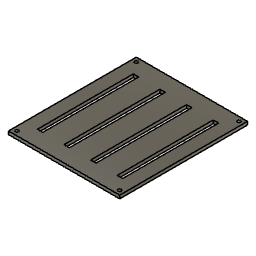
Quadrotor_controller_case_lid_plain (Autodesk Fusion 360 design; units mm, degrees)
Autodesk Fusion 360 part; units mm, degrees
sketch "Sketch1" plane through (0, 0, 0) normal (0, 0, 1) x (1, 0, 0)
  line L0 (-52.2, -60) -> (52.2, -60)
  line L1 (52.2, -60) -> (52.2, 60)
  line L2 (52.2, 60) -> (-52.2, 60)
  line L3 (-52.2, 60) -> (-52.2, -60)
  dimension "d1" = 104.4
  dimension "d2" = 120
  dimension "d3" = 60
  dimension "d4" = 52.2
  constraint horizontal L0
  constraint vertical L1
  constraint horizontal L2
  constraint vertical L3
  measures "d1" distance of L0.start L0.end
  measures "d2" distance of L0.start L2.end
  measures "d3" vertical distance of origin L0.start
  measures "d4" horizontal distance of origin L0.start
extrude "Extrude1" add sketch "Sketch1" along normal blind 3
sketch "Sketch2" plane through (0, 0, 3) normal (0, 0, 1) x (-1, 0, 0)
  line L0 (52.2, -60) -> (52.2, 60)
  line L1 (52.2, 60) -> (-52.2, 60)
  line L2 (-52.2, 60) -> (-52.2, -60)
  line L3 (-52.2, -60) -> (52.2, -60)
  circle A0 centre (-48.2, -56) radius 1.5
  circle A1 centre (48.2, -56) radius 1.5
  circle A2 centre (48.2, 56) radius 1.5
  circle A3 centre (-48.2, 56) radius 1.5
  dimension "d7" = 3
  dimension "d8" = 3
  dimension "d9" = 3
  dimension "d10" = 3
  dimension "d11" = 4
  dimension "d12" = 4
  dimension "d13" = 4
  dimension "d14" = 4
  dimension "d15" = 4
  dimension "d16" = 4
  dimension "d17" = 4
  dimension "d18" = 4
  measures "d7" diameter of A0
  measures "d8" diameter of A1
  measures "d9" diameter of A3
  measures "d10" diameter of A2
  measures "d11" distance of L2 A0.centre
  measures "d12" distance of L3 A0.centre
  measures "d13" distance of L3 A1.centre
  measures "d14" distance of L0 A1.centre
  measures "d15" distance of L1 A2.centre
  measures "d16" distance of L0 A2.centre
  measures "d17" distance of L2 A3.centre
  measures "d18" distance of L1 A3.centre
hole "Hole1" at (-48.2, 56, 3) at (48.2, 56, 3) at (48.2, -56, 3) at (-48.2, -56, 3) direction (0, 0, -1) diameter 3 depth 3 tip angle 118
sketch "Sketch4" plane through (0, 0, 3) normal (0, 0, 1) x (-1, 0, 0)
  circle A0 centre (-48.2, 56) radius 1.5
  circle A1 centre (48.2, -56) radius 1.5
  circle A2 centre (-48.2, -56) radius 1.5
  circle A3 centre (48.2, 56) radius 1.5
  line L0 (52.2, -60) -> (52.2, 60)
  line L1 (52.2, 60) -> (-52.2, 60)
  line L2 (-52.2, 60) -> (-52.2, -60)
  line L3 (-52.2, -60) -> (52.2, -60)
  line L4 (40, -45) -> (35, -45)
  line L5 (35, -45) -> (35, 45)
  line L6 (35, 45) -> (40, 45)
  line L7 (40, 45) -> (40, -45)
  line L8 (10, -45) -> (10, 45)
  line L9 (10, 45) -> (15, 45)
  line L10 (15, 45) -> (15, -45)
  line L11 (15, -45) -> (10, -45)
  line L12 (-15, -45) -> (-15, 45)
  line L13 (-15, 45) -> (-10, 45)
  line L14 (-10, 45) -> (-10, -45)
  line L15 (-10, -45) -> (-15, -45)
  line L16 (-40, -45) -> (-40, 45)
  line L17 (-40, 45) -> (-35, 45)
  line L18 (-35, 45) -> (-35, -45)
  line L19 (-35, -45) -> (-40, -45)
  dimension "d39" = -75
  dimension "d40" = 0
  dimension "d41" = 5
  dimension "d42" = 90
  dimension "d43" = 40
  dimension "d44" = 45
  constraint horizontal L4
  constraint vertical L5
  constraint horizontal L6
  constraint vertical L7
  measures "d41" distance of L4.start L4.end
  measures "d42" distance of L4.start L6.end
  measures "d43" distance of origin L7
  measures "d44" distance of origin L4
extrude "Extrude2" cut sketch "Sketch4" against normal blind 3 contours L4 L5 L6 L7 | L8 L9 L10 L11 | L12 L13 L14 L15 | L16 L17 L18 L19
sketch "Sketch6" plane through (0, 0, 3) normal (0, 0, 1) x (-1, 0, 0)
  line L0 (10, 45) -> (15, 45)
  line L1 (15, 45) -> (15, -45)
  line L2 (15, -45) -> (10, -45)
  line L3 (10, -45) -> (10, 45)
  line L4 (-15, 45) -> (-10, 45)
  line L5 (-10, 45) -> (-10, -45)
  line L6 (-10, -45) -> (-15, -45)
  line L7 (-15, -45) -> (-15, 45)
  line L8 (35, -45) -> (35, 45)
  line L9 (35, 45) -> (40, 45)
  line L10 (40, 45) -> (40, -45)
  line L11 (40, -45) -> (35, -45)
  line L12 (-40, 45) -> (-35, 45)
  line L13 (-35, 45) -> (-35, -45)
  line L14 (-35, -45) -> (-40, -45)
  line L15 (-40, -45) -> (-40, 45)
  circle A0 centre (-48.2, 56) radius 1.5
  circle A1 centre (48.2, -56) radius 1.5
  circle A2 centre (-48.2, -56) radius 1.5
  circle A3 centre (48.2, 56) radius 1.5
  line L16 (52.2, -60) -> (52.2, 60)
  line L17 (52.2, 60) -> (-52.2, 60)
  line L18 (-52.2, 60) -> (-52.2, -60)
  line L19 (-52.2, -60) -> (52.2, -60)
  line L20 (-15, 25) -> (15, 25)
  line L21 (15, 25) -> (15, -25)
  line L22 (15, -25) -> (-15, -25)
  line L23 (-15, -25) -> (-15, 25)
  line L24 (-15, 25) -> (15, -25) construction
  line L25 (15, 25) -> (-15, -25) construction
  line L26 (40, -8) -> (35, -8)
  line L27 (35, -8) -> (35, 8)
  line L28 (35, 8) -> (40, 8)
  line L29 (40, 8) -> (40, -8)
  line L30 (-35, -8) -> (-40, -8)
  line L31 (-40, -8) -> (-40, 8)
  line L32 (-40, 8) -> (-35, 8)
  line L33 (-35, 8) -> (-35, -8)
  dimension "d49" = 50
  dimension "d56" = 8
  dimension "d57" = 16
  dimension "d58" = 8
  dimension "d59" = 16
  constraint horizontal L20
  constraint perpendicular L20 L21
  constraint parallel L20 L22
  constraint parallel L21 L23
  constraint coincident L24 origin
  constraint coincident L25 origin
  constraint coincident L7 L20.start
  constraint horizontal L26
  constraint vertical L27
  constraint horizontal L28
  constraint vertical L29
  constraint coincident L8 L27.end
  constraint coincident L10 L26.start
  constraint horizontal L30
  constraint vertical L31
  constraint horizontal L32
  constraint vertical L33
  constraint coincident L15 L31.end
  constraint coincident L13 L30.start
  measures "d49" distance of L20.end L21.end
  measures "d56" vertical distance of origin L27.end
  measures "d57" vertical distance of L26.start L27.end
  measures "d58" vertical distance of origin L31.end
  measures "d59" vertical distance of L30.start L31.end
extrude "Extrude3" [rolled back] along distance -3 taper angle 0
sketch "Sketch5" plane through (0, 0, 3) normal (0, 0, 1) x (-1, 0, 0)
  line L0 (10, 45) -> (15, 45)
  line L1 (15, 45) -> (15, 25)
  line L2 (15, -45) -> (10, -45)
  line L3 (10, 25) -> (10, 45)
  line L4 (-15, 45) -> (-10, 45)
  line L5 (-10, -25) -> (-10, -45)
  line L6 (-10, -45) -> (-15, -45)
  line L7 (-15, -45) -> (-15, -25)
  line L8 (35, 8) -> (35, 45)
  line L9 (35, 45) -> (40, 45)
  line L10 (40, 45) -> (40, 8)
  line L11 (40, -45) -> (35, -45)
  line L12 (-40, 45) -> (-35, 45)
  line L13 (-35, 45) -> (-35, 8)
  line L14 (-35, -45) -> (-40, -45)
  line L15 (-40, 8) -> (-40, 45)
  circle A0 centre (-48.2, 56) radius 1.5
  circle A1 centre (48.2, -56) radius 1.5
  circle A2 centre (-48.2, -56) radius 1.5
  circle A3 centre (48.2, 56) radius 1.5
  line L16 (52.2, -60) -> (52.2, 60)
  line L17 (52.2, 60) -> (-52.2, 60)
  line L18 (-52.2, 60) -> (-52.2, -60)
  line L19 (-52.2, -60) -> (52.2, -60)
  circle A4 centre (0, 0) radius 11.25
  circle A5 centre (0, 0) radius 15
  line L20 (15, 25) -> (10, 25)
  line L21 (-15, -25) -> (-10, -25)
  line L22 (10, -25) -> (15, -25)
  line L23 (15, -25) -> (15, -45)
  line L24 (10, -45) -> (10, -25)
  line L25 (-10, 25) -> (-15, 25)
  line L26 (-15, 25) -> (-15, 45)
  line L27 (-10, 45) -> (-10, 25)
  line L28 (-35, 8) -> (-40, 8)
  line L29 (40, 8) -> (35, 8)
  line L30 (35, -8) -> (40, -8)
  line L31 (40, -8) -> (40, -45)
  line L32 (35, -45) -> (35, -8)
  line L33 (-40, -8) -> (-35, -8)
  line L34 (-35, -8) -> (-35, -45)
  line L35 (-40, -45) -> (-40, -8)
  dimension "d47" = 22.5
  dimension "d48" = 30
  constraint coincident A4.centre A5.centre
  measures "d47" diameter of A4
  measures "d48" diameter of A5
extrude "Extrude4" [rolled back] along distance 30 taper angle 0
fillet "Fillet1" [rolled back] radius 6
chamfer "Chamfer1" [rolled back] distance 0.5
sketch "Sketch7" plane through (0, 0, 0) normal (0, 1, 0) x (1, 0, 0)
  circle A0 centre (-0.0436, -26) radius 1.5
  dimension "d61" = 26
  dimension "d62" = 3
  measures "d61" vertical distance of origin A0.centre
  measures "d62" diameter of A0
hole "Hole3" [rolled back] hole depth 17 hole diameter 3 tip angle 118
thread "Thread1" [rolled back]
pattern_circular "C-Pattern1" [rolled back] total angle 360
hole "Hole4" [rolled back] hole depth 3 hole diameter 16 tip angle 118
sketch "Sketch8" plane through (0, 0, 0) normal (0, 0, -1) x (1, 0, 0)
  circle A0 centre (0, 0) radius 8
  line L0 (40, -8) -> (40, -45)
  line L1 (40, -45) -> (35, -45)
  line L2 (35, -45) -> (35, -8)
  line L3 (35, -8) -> (40, -8)
  line L4 (-10, -25) -> (-10, -45)
  line L5 (-10, -45) -> (-15, -45)
  line L6 (-15, -45) -> (-15, -25)
  line L7 (-15, -25) -> (-10, -25)
  line L8 (-35, -8) -> (-35, -45)
  line L9 (-35, -45) -> (-40, -45)
  line L10 (-40, -45) -> (-40, -8)
  line L11 (-40, -8) -> (-35, -8)
  line L12 (10, 25) -> (10, 45)
  line L13 (10, 45) -> (15, 45)
  line L14 (15, 45) -> (15, 25)
  line L15 (15, 25) -> (10, 25)
  line L16 (-10, 25) -> (-15, 25)
  line L17 (-15, 25) -> (-15, 45)
  line L18 (-15, 45) -> (-10, 45)
  line L19 (-10, 45) -> (-10, 25)
  line L20 (10, -25) -> (15, -25)
  line L21 (15, -25) -> (15, -45)
  line L22 (15, -45) -> (10, -45)
  line L23 (10, -45) -> (10, -25)
  line L24 (-35, 8) -> (-40, 8)
  line L25 (-40, 8) -> (-40, 45)
  line L26 (-40, 45) -> (-35, 45)
  line L27 (-35, 45) -> (-35, 8)
  line L28 (40, 8) -> (35, 8)
  line L29 (35, 8) -> (35, 45)
  line L30 (35, 45) -> (40, 45)
  line L31 (40, 45) -> (40, 8)
  circle A1 centre (48.2, 56) radius 1.5
  circle A2 centre (-48.2, -56) radius 1.5
  circle A3 centre (48.2, -56) radius 1.5
  circle A4 centre (-48.2, 56) radius 1.5
  line L32 (-52.2, 60) -> (-52.2, -60)
  line L33 (-52.2, -60) -> (52.2, -60)
  line L34 (52.2, -60) -> (52.2, 60)
  line L35 (52.2, 60) -> (-52.2, 60)
  line L36 (-21.595, 55.595) -> (21.595, 55.595)
  line L37 (21.595, 55.595) -> (21.595, 12.405)
  line L38 (21.595, 12.405) -> (-21.595, 12.405)
  line L39 (-21.595, 12.405) -> (-21.595, 55.595)
  line L40 (-25.4, -12.405) -> (25.4, -12.405)
  line L41 (25.4, -12.405) -> (25.4, -55.595)
  line L42 (25.4, -55.595) -> (-25.4, -55.595)
  line L43 (-25.4, -55.595) -> (-25.4, -12.405)
  line L44 (-19.055, 53.055) -> (19.055, 53.055)
  line L45 (19.055, 53.055) -> (19.055, 14.945)
  line L46 (19.055, 14.945) -> (-19.055, 14.945)
  line L47 (-19.055, 14.945) -> (-19.055, 53.055)
  line L48 (-22.86, -14.945) -> (22.86, -14.945)
  line L49 (22.86, -14.945) -> (22.86, -53.055)
  line L50 (22.86, -53.055) -> (-22.86, -53.055)
  line L51 (-22.86, -53.055) -> (-22.86, -14.945)
  dimension "d71" = 43.19
  dimension "d72" = 43.19
  dimension "d73" = 50.8
  dimension "d74" = 43.19
  dimension "d75" = 2.54
  dimension "d76" = 2.54
  dimension "d77" = 2.54
  dimension "d78" = 2.54
  dimension "d79" = 2.54
  dimension "d80" = 2.54
  dimension "d81" = 2.54
  dimension "d82" = 2.54
  dimension "d83" = 25.4
  dimension "d84" = 21.595
  dimension "d85" = 4.405
  dimension "d86" = 4.405
  constraint horizontal L36
  constraint vertical L37
  constraint horizontal L38
  constraint vertical L39
  constraint horizontal L40
  constraint vertical L41
  constraint horizontal L42
  constraint vertical L43
  constraint horizontal L44
  constraint vertical L45
  constraint horizontal L46
  constraint vertical L47
  constraint horizontal L48
  constraint vertical L49
  constraint horizontal L50
  constraint vertical L51
  measures "d71" distance of L36.start L36.end
  measures "d72" distance of L36.end L37.end
  measures "d73" distance of L40.start L40.end
  measures "d74" distance of L40.end L41.end
  measures "d75" distance of L39 L47
  measures "d76" distance of L36 L44
  measures "d77" distance of L38 L46
  measures "d78" distance of L37 L45
  measures "d79" distance of L41 L49
  measures "d80" distance of L43 L51
  measures "d81" distance of L42 L50
  measures "d82" distance of L40 L48
  measures "d83" horizontal distance of A0.centre L40.start
  measures "d84" horizontal distance of A0.centre L38.end
  measures "d85" distance of L35 L36
  measures "d86" distance of L33 L42
hole "Hole5" [rolled back] hole depth 3 hole diameter 3 tip angle 118
